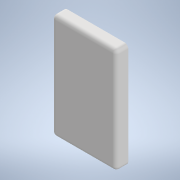
# Autodesk Inventor part: kris
Saved by Autodesk Inventor 2022 (Build 260153000, 153)
## iProperties
Created: 2023-05-24
Part Number: kris
Material: Типовые
Document SubType Name: Modeling
Designer: korsh624
Density: 1 g/cm^3
Appearance: По умолчанию
Author: korsh624
Autodesk Inventor part; units mm, degrees
ref_plane "YZ Plane" through (0, 0, 0) normal (1, 0, 0) x (0, 1, 0)
ref_plane "XZ Plane" through (0, 0, 0) normal (0, 1, 0) x (-1, 0, 0)
ref_plane "XY Plane" through (0, 0, 0) normal (0, 0, 1) x (1, 0, 0)
sketch "Эскиз1" plane through (0, 0, 0) normal (0, 0, 1) x (1, 0, 0)
  line L0 (5, 13) -> (5, 207.8488) projected
  arc A0 (13, 215.8488) -> (5, 207.8488) centre (13, 207.8488) ccw projected
  line L1 (13, 215.8488) -> (122.6512, 215.8488) projected
  arc A1 (130.6512, 207.8488) -> (122.6512, 215.8488) centre (122.6512, 207.8488) ccw projected
  line L2 (130.6512, 207.8488) -> (130.6512, 13) projected
  arc A2 (122.6512, 5) -> (130.6512, 13) centre (122.6512, 13) ccw projected
  line L3 (13, 5) -> (122.6512, 5) projected
  arc A3 (5, 13) -> (13, 5) centre (13, 13) ccw projected
  arc A4 (127.6512, 0) -> (135.6512, 8) centre (127.6512, 8) ccw projected
  line L4 (135.6512, 8) -> (135.6512, 212.8488) projected
  arc A5 (135.6512, 212.8488) -> (127.6512, 220.8488) centre (127.6512, 212.8488) ccw projected
  line L5 (127.6512, 220.8488) -> (8, 220.8488) projected
  arc A6 (8, 220.8488) -> (0, 212.8488) centre (8, 212.8488) ccw projected
  line L6 (0, 8) -> (0, 212.8488) projected
  arc A7 (0, 8) -> (8, 0) centre (8, 8) ccw projected
  line L7 (127.6512, 0) -> (8, 0) projected
  point P0 (0, 0)
extrude "Выдавливание1" add sketch "Эскиз1" along normal blind 20
sketch "Эскиз2" plane through (0, 0, 20) normal (0, 0, 1) x (1, 0, 0)
  line L0 (8, 0) -> (127.6512, 0) projected
  arc A0 (127.6512, 0) -> (135.6512, 8) centre (127.6512, 8) ccw projected
  line L1 (135.6512, 8) -> (135.6512, 212.8488) projected
  arc A1 (135.6512, 212.8488) -> (127.6512, 220.8488) centre (127.6512, 212.8488) ccw projected
  line L2 (127.6512, 220.8488) -> (8, 220.8488) projected
  arc A2 (8, 220.8488) -> (0, 212.8488) centre (8, 212.8488) ccw projected
  line L3 (0, 212.8488) -> (0, 8) projected
  arc A3 (0, 8) -> (8, 0) centre (8, 8) ccw projected
  arc A4 (5, 13) -> (13, 5) centre (13, 13) ccw projected
  line L4 (5, 13) -> (5, 207.8488) projected
  arc A5 (13, 215.8488) -> (5, 207.8488) centre (13, 207.8488) ccw projected
  line L5 (13, 215.8488) -> (122.6512, 215.8488) projected
  arc A6 (130.6512, 207.8488) -> (122.6512, 215.8488) centre (122.6512, 207.8488) ccw projected
  line L6 (130.6512, 207.8488) -> (130.6512, 13) projected
  arc A7 (122.6512, 5) -> (130.6512, 13) centre (122.6512, 13) ccw projected
  line L7 (122.6512, 5) -> (13, 5) projected
  point P0 (0, 0)
extrude "Выдавливание2" add sketch "Эскиз2" along normal blind 5 contours A3 L3 A2 L2 A1 L1 A0 L0 | L4 A5 L5 A6 L6 A7 L7 A4
fillet "Сопряжение1" radius 8 16 edges at (133.308, 218.5056, 25) (67.8256, 220.8488, 25) (2.3431, 218.5056, 25) (0, 110.4244, 25) (2.3431, 2.3431, 25) (67.8256, 0, 25) (133.308, 2.3431, 25) (135.6512, 110.4244, 25) (128.308, 7.3431, 20) (67.8256, 5, 20) (7.3431, 7.3431, 20) (5, 110.4244, 20) (7.3431, 213.5056, 20) (67.8256, 215.8488, 20) (128.308, 213.5056, 20) (130.6512, 110.4244, 20)
